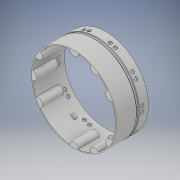
# Autodesk Inventor part: Than_new
Saved by Autodesk Inventor 2019 (Build 230136000, 136)
## iProperties
Created: 2021-01-14
Part Number: Than_new
Material: Generic
Document SubType Name: Modeling
Designer: Admin
Density: 1 g/cm^3
Appearance: Default
Author: Admin
Autodesk Inventor part; units mm, degrees
ref_plane "YZ Plane" through (0, 0, 0) normal (1, 0, 0) x (0, 1, 0)
ref_plane "XZ Plane" through (0, 0, 0) normal (0, 1, 0) x (-1, 0, 0)
ref_plane "XY Plane" through (0, 0, 0) normal (0, 0, 1) x (1, 0, 0)
sketch "Sketch1" plane through (0, 0, 0) normal (0, 0, 1) x (1, 0, 0)
  circle A0 centre (0, 0) radius 200
  circle A1 centre (0, 0) radius 195
  dimension "d0" = 400
  dimension "d1" = 390
  constraints: 2 centre point, 2 coincident
  measures "d0" diameter of A0
  measures "d1" diameter of A1
extrude "Extrusion1" add sketch "Sketch1" along normal blind 150
ref_plane "Work Plane1" through (0, 0, 50) normal (0, 0, 1) x (1, 0, 0)
sketch "Sketch2" plane through (0, 0, 50) normal (0, 0, 1) x (1, 0, 0)
  circle A0 centre (0, 0) radius 200
  circle A1 centre (0, 0) radius 197.5
  dimension "d5" = 395
  constraints: 2 centre point, 2 coincident
  measures "d5" diameter of A1
extrude "Extrusion2" cut sketch "Sketch2" along normal mid plane 10
fillet "Fillet1" radius 2 4 edges at (-200, 0, 45) (-197.5, 0, 45) (-200, 0, 55) (-197.5, 0, 55)
sketch "Sketch3" plane through (0, 0, 150) normal (0, 0, 1) x (1, 0, 0)
  arc A0 (173.6513, 88.7144) -> (163.6545, 106.0292) centre (0, 0) ccw
  arc A1 (106.0292, 163.6545) -> (88.7144, 173.6513) centre (0, 0) ccw
  arc A2 (9.9967, 194.7436) -> (-9.9967, 194.7436) centre (0, 0) ccw
  arc A3 (-163.6545, 106.0292) -> (-173.6513, 88.7144) centre (0, 0) ccw
  arc A4 (-194.7436, 9.9967) -> (-194.7436, -9.9967) centre (0, 0) ccw
  arc A5 (-173.6513, -88.7144) -> (-163.6545, -106.0292) centre (0, 0) ccw
  arc A6 (-9.9967, -194.7436) -> (9.9967, -194.7436) centre (0, 0) ccw
  arc A7 (88.7144, -173.6513) -> (106.0292, -163.6545) centre (0, 0) ccw
  arc A8 (163.6545, -106.0292) -> (173.6513, -88.7144) centre (0, 0) ccw
  arc A9 (177.9736, -79.6895) -> (157.9999, -114.2849) centre (168.875, -97.5) ccw
  arc A10 (114.2849, -157.9999) -> (79.6895, -177.9736) centre (97.5, -168.875) ccw
  arc A11 (19.9737, -193.9744) -> (-19.9737, -193.9744) centre (0, -195) ccw
  arc A12 (157.9999, 114.2849) -> (177.9736, 79.6895) centre (168.875, 97.5) ccw
  arc A13 (79.6895, 177.9736) -> (114.2849, 157.9999) centre (97.5, 168.875) ccw
  arc A14 (-19.9852, 193.9732) -> (19.9852, 193.9732) centre (0, 194.7436) ccw
  arc A15 (-193.9744, -19.9737) -> (-193.9744, 19.9737) centre (-195, 0) ccw
  arc A16 (-177.9736, 79.6895) -> (-157.9999, 114.2849) centre (-168.875, 97.5) ccw
  arc A17 (-157.9999, -114.2849) -> (-177.9736, -79.6895) centre (-168.875, -97.5) ccw
  arc A18 (79.6895, -177.9736) -> (114.2849, -157.9999) centre (0, 0) ccw
  arc A19 (157.9999, -114.2849) -> (177.9736, -79.6895) centre (0, 0) ccw
  arc A20 (177.9736, 79.6895) -> (157.9999, 114.2849) centre (0, 0) ccw
  arc A21 (114.2849, 157.9999) -> (79.6895, 177.9736) centre (0, 0) ccw
  arc A22 (19.9852, 193.9732) -> (-19.9852, 193.9732) centre (0, 0) ccw
  arc A23 (-157.9999, 114.2849) -> (-177.9736, 79.6895) centre (0, 0) ccw
  arc A24 (-193.9744, 19.9737) -> (-193.9744, -19.9737) centre (0, 0) ccw
  arc A25 (-177.9736, -79.6895) -> (-157.9999, -114.2849) centre (0, 0) ccw
  arc A26 (-19.9737, -193.9744) -> (19.9737, -193.9744) centre (0, 0) ccw
  dimension "d22" = 40
  dimension "d23" = 40
  dimension "d24" = 40
  dimension "d25" = 40
  dimension "d26" = 40
  dimension "d27" = 40
  dimension "d28" = 40
  dimension "d29" = 40
  dimension "d30" = 40
  constraints: 54 point on circle, 27 centre point, 2 coincident
  measures "d22" diameter of A9
  measures "d23" diameter of A10
  measures "d24" diameter of A11
  measures "d25" diameter of A12
  measures "d26" diameter of A13
  measures "d27" diameter of A14
  measures "d28" diameter of A15
  measures "d29" diameter of A16
  measures "d30" diameter of A17
extrude "Extrusion3" add sketch "Sketch3" against normal blind 100
sketch "Sketch4" plane through (0, 0, 50) normal (0, 0, 1) x (1, 0, 0)
  line L0 (185, 0) -> (185, 10)
  line L1 (185, 10) -> (195, 10)
  line L2 (195, 10) -> (195, 0)
  line L3 (185, 0) -> (185, -10)
  line L4 (185, -10) -> (195, -10)
  line L5 (195, -10) -> (195, 0)
  line L6 (-92.5, 160.2147) -> (-101.1603, 155.2147)
  line L7 (-101.1603, 155.2147) -> (-106.1603, 163.875)
  line L8 (-106.1603, 163.875) -> (-97.5, 168.875)
  line L9 (-92.5, 160.2147) -> (-83.8397, 165.2147)
  line L10 (-83.8397, 165.2147) -> (-88.8397, 173.875)
  line L11 (-88.8397, 173.875) -> (-97.5, 168.875)
  line L12 (-92.5, -160.2147) -> (-83.8397, -165.2147)
  line L13 (-83.8397, -165.2147) -> (-88.8397, -173.875)
  line L14 (-88.8397, -173.875) -> (-97.5, -168.875)
  line L15 (-92.5, -160.2147) -> (-101.1603, -155.2147)
  line L16 (-101.1603, -155.2147) -> (-106.1603, -163.875)
  line L17 (-106.1603, -163.875) -> (-97.5, -168.875)
  line L18 (-101.1603, 155.2147) -> (-83.8397, 165.2147)
  line L19 (-88.8397, 173.875) -> (-106.1603, 163.875)
  circle A0 centre (-95, -164.5448) radius 1.5
  circle A1 centre (190, 0) radius 1.5
  point P0 (0, 0)
  point P1 (173.6513, 88.7144)
  point P2 (173.6513, -88.7144)
  point P3 (0, 0)
  dimension "d18" = 360
  dimension "d38" = 3
  constraints: 40 end point, 2 centre point, 1 coincident, 1 collinear, 1 parallel, 37 other
  measures "d38" diameter of A0
extrude "Extrusion4" add sketch "Sketch4" along normal blind 10 contours L0 L1 L2 L5 L4 L3 | L12 L13 L14 L17 L16 L15 | A0 | A1
sketch "Sketch5" plane through (0, 0, 0) normal (1, 0, 0) x (0, 1, 0)
  line L0 (-79.6895, 150) -> (79.6895, 150) projected
  circle A0 centre (12.75, 29) radius 8
  circle A1 centre (-12.75, 29) radius 8
  point P0 (0, 0)
  dimension "d32" = 16
  constraints: 2 centre point
  measures "d32" diameter of A0
extrude "Extrusion5" cut sketch "Sketch5" against normal blind 1000
pattern_circular "Circular Pattern1" count 10 over 360 about axis through (0, 0, 0) along (0, 0, 1) of "Extrusion5"
extrude "Extrusion6" cut sketch "Sketch4" along normal blind 5 contours A0
extrude "Extrusion7" cut sketch "Sketch4" along normal blind 5 contours A1
body "Solid1"
